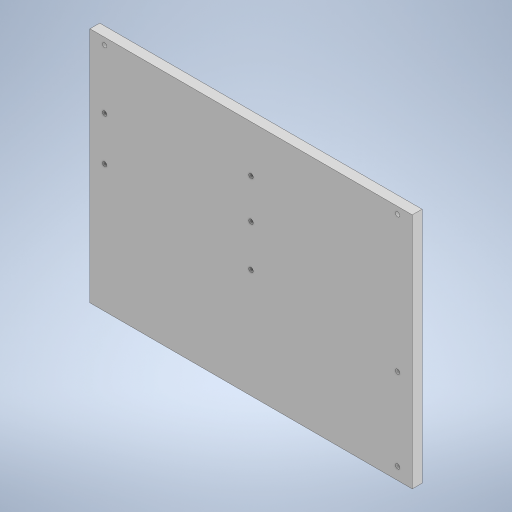
# Autodesk Inventor part: Validation_jig_top
Saved by Autodesk Inventor 2023 (Build 270158000, 158)
## iProperties
Created: 2023-02-22
Part Number: Validation_jig_top
Material: Générique
Document SubType Name: Modeling
Designer: jfcoe
Density: 1 g/cm^3
Appearance: Par défaut
Author: jfcoe
Autodesk Inventor part; units mm, degrees
ref_plane "YZ Plane" through (0, 0, 0) normal (1, 0, 0) x (0, 1, 0)
ref_plane "XZ Plane" through (0, 0, 0) normal (0, 1, 0) x (-1, 0, 0)
ref_plane "XY Plane" through (0, 0, 0) normal (0, 0, 1) x (1, 0, 0)
sketch "Esquisse1" plane through (0, 0, 0) normal (0, 0, 1) x (1, 0, 0)
  line L0 (0, 0) -> (220, 0)
  line L1 (220, 0) -> (220, -162)
  line L2 (220, -162) -> (0, -162)
  line L3 (0, -162) -> (0, 0)
  dimension "d0" = 220
  dimension "d1" = 162
  constraints: 8 end point, 2 parallel, 1 horizontal, 1 perpendicular
  measures "d0" distance of L1.end L2.end
  measures "d1" distance of L0.end L1.end
extrude "Extrusion1" add sketch "Esquisse1" against normal blind 6.7
sketch "Esquisse2" plane through (0, 0, 0) normal (0, 0, 1) x (1, 0, 0)
  circle A0 centre (10, -4.675) radius 1.524
  circle A1 centre (110, -32) radius 1.524
  circle A2 centre (210, -4.675) radius 1.524
  circle A3 centre (210, -97.675) radius 1.524
  circle A4 centre (110, -87.5) radius 1.524
  circle A5 centre (10, -45) radius 1.524
  circle A6 centre (110, -59) radius 1.524
  circle A7 centre (210, -153.675) radius 1.524
  line L0 (220, 0) -> (0, 0) projected
  line L1 (0, 0) -> (0, -162) projected
  line L2 (220, -162) -> (220, 0) projected
  circle A8 centre (10, -75) radius 1.524
  dimension "d4" = 3.048
  dimension "d5" = 4.675
  dimension "d6" = 10
  dimension "d7" = 10
  dimension "d9" = 10
  dimension "d10" = 10
  dimension "d11" = 10
  dimension "d15" = 32
  dimension "d16" = 27
  dimension "d17" = 28.5
  dimension "d18" = 4.675
  dimension "d19" = 93
  dimension "d20" = 56
  dimension "d21" = 40.325
  dimension "d22" = 10
  dimension "d26" = 110
  dimension "d27" = 110
  dimension "d28" = 110
  dimension "d29" = 30
  constraints: 9 centre point, 8 equal radius
  measures "d4" diameter of A0
  measures "d5" distance from line of L0 A0.centre
  measures "d6" distance from line of L1 A0.centre
  measures "d7" distance from line of L1 A5.centre
  measures "d9" distance from line of L2 A2.centre
  measures "d10" distance from line of L2 A3.centre
  measures "d11" distance from line of L2 A7.centre
  measures "d15" distance from line of L0 A1.centre
  measures "d16" distance of A6.centre A1.centre
  measures "d17" distance of A4.centre A6.centre
  measures "d18" distance from line of L0 A2.centre
  measures "d19" distance of A2.centre A3.centre
  measures "d20" distance of A3.centre A7.centre
  measures "d21" distance of A5.centre A0.centre
  measures "d22" distance from line of L1 A8.centre
  measures "d26" distance from line of L1 A1.centre
  measures "d27" distance from line of L1 A6.centre
  measures "d28" distance from line of L1 A4.centre
  measures "d29" distance of A8.centre A5.centre
extrude "Extrusion2" cut sketch "Esquisse2" against normal through all
